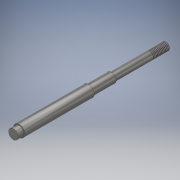
# Autodesk Inventor part: AxeArriere
Saved by Autodesk Inventor 2019 (Build 230136000, 136)
## iProperties
Created: 2019-07-30
Part Number: AxeArriere
Material: Acier inoxydable
Document SubType Name: Modeling
Designer: Sébastien DI MERCURIO
Mass: 8.25611 g
Surface Area: 7.44557 cm^2
Volume: 1.03201 cm^3
Density: 8 g/cm^3
Appearance: Semi-poli
Author: Sébastien DI MERCURIO
Autodesk Inventor part; units mm, degrees
ref_plane "YZ Plane" through (0, 0, 0) normal (1, 0, 0) x (0, 1, 0)
ref_plane "XZ Plane" through (0, 0, 0) normal (0, 1, 0) x (-1, 0, 0)
ref_plane "XY Plane" through (0, 0, 0) normal (0, 0, 1) x (1, 0, 0)
sketch "Esquisse1" plane through (0, 0, 0) normal (0, 0, 1) x (1, 0, 0)
  circle A0 centre (0, 0) radius 3
  dimension "d0" = 6
  constraints: 1 centre point, 1 coincident
  measures "d0" diameter of A0
extrude "Extrusion1" add sketch "Esquisse1" along normal blind 36.5
sketch "Esquisse2" plane through (0, 0, 36.5) normal (0, 0, 1) x (1, 0, 0)
  circle A0 centre (0, 0) radius 2.5
  dimension "d3" = 5
  constraints: 1 centre point, 1 coincident
  measures "d3" diameter of A0
extrude "Extrusion2" add sketch "Esquisse2" along normal blind 3
sketch "Esquisse3" plane through (0, 0, 0) normal (0, 0, -1) x (-1, 0, 0)
  circle A0 centre (0, 0) radius 2.5
  dimension "d6" = 5
  constraints: 1 centre point, 1 coincident
  measures "d6" diameter of A0
extrude "Extrusion3" add sketch "Esquisse3" along normal blind 12
sketch "Esquisse4" plane through (0, 0, -12) normal (0, 0, -1) x (-1, 0, 0)
  circle A0 centre (0, 0) radius 2
  dimension "d9" = 4
  constraints: 1 centre point, 1 coincident
  measures "d9" diameter of A0
extrude "Extrusion4" add sketch "Esquisse4" along normal blind 29
thread "Filetage1" size "M4x0.7" class "6g" standard "ANSI Metric M Profile" length 9
fillet "Congé1" radius 0.5 1 edges at (2, 0, -41)
